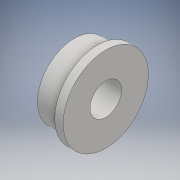
# Autodesk Inventor part: bearing_683
Saved by Autodesk Inventor 2017 (Build 210142000, 142)
## iProperties
Part Number: bearing_683
Material: 一般
Document SubType Name: Modeling
Designer: sktom
Density: 1 g/cm^3
Appearance: 既定
Author: sktom
Autodesk Inventor part; units mm, degrees
ref_plane "YZ Plane" through (0, 0, 0) normal (1, 0, 0) x (0, 1, 0)
ref_plane "XZ Plane" through (0, 0, 0) normal (0, 1, 0) x (-1, 0, 0)
ref_plane "XY Plane" through (0, 0, 0) normal (0, 0, 1) x (1, 0, 0)
sketch "スケッチ1" plane through (0, 0, 0) normal (0, 0, 1) x (1, 0, 0)
  line L0 (0, 1.5) -> (3, 1.5)
  line L1 (3, 1.5) -> (3, 4.05)
  line L2 (3, 4.05) -> (2.2, 4.05)
  line L3 (2.2, 4.05) -> (2.2, 3.5)
  line L4 (2.2, 3.5) -> (0, 3.5)
  line L5 (0, 3.5) -> (0, 1.5)
  line L6 (0, 0) -> (3, 0) construction
  dimension "d0" = 1.5
  dimension "d1" = 3.5
  dimension "d2" = 0.8
  dimension "d3" = 3
  dimension "d4" = 4.05
  constraints: 14 end point, 5 perpendicular, 2 horizontal, 1 vertical alignment
  measures "d0" distance from line of L6.start L0
  measures "d1" distance from line of L6.start L4
  measures "d2" distance of L1.end L2.end
  measures "d3" distance of L0.start L0.end
  measures "d4" distance from line of L6.start L2
revolve "回転1" add sketch "スケッチ1" angle 360 about axis through (0, 0, 0) along (1, 0, 0)
